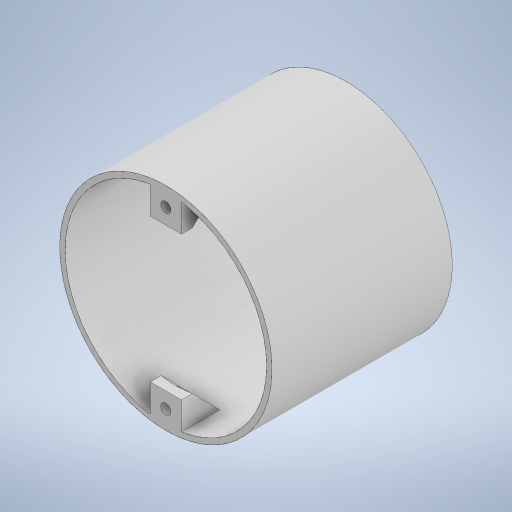
# Autodesk Inventor part: LensMount_mount
Saved by Autodesk Inventor 2023 (Build 270158000, 158)
## iProperties
Created: 2022-10-30
Part Number: LensMount_mount
Material: Generic
Document SubType Name: Modeling
Designer: Piotr
Density: 1 g/cm^3
Appearance: Default
Author: Piotr
Autodesk Inventor part; units mm, degrees
ref_plane "YZ Plane" through (0, 0, 0) normal (1, 0, 0) x (0, 1, 0)
ref_plane "XZ Plane" through (0, 0, 0) normal (0, 1, 0) x (-1, 0, 0)
sketch "Sketch1" plane through (0, 0, 0) normal (0, 0, 1) x (1, 0, 0)
  circle A0 centre (0, 0) radius 32.25
  circle A1 centre (0, 0) radius 34
  line L0 (0, 0) -> (34, 0) construction
  line L1 (0, 0) -> (30.0202, 15.962) construction
  circle A2 centre (0, 0) radius 30.7
  line L2 (0, 0) -> (26.7199, 15.1174) construction
  line L3 (0, 0) -> (27.4745, 13.6983) construction
  line L4 (28.069, 15.8807) -> (29.5921, 16.7424) construction
  line L5 (28.8616, 14.3899) -> (30.4278, 15.1707) construction
  line L6 (27.4745, 13.6983) -> (28.8616, 14.3899)
  line L7 (26.7199, 15.1174) -> (28.069, 15.8807)
  line L8 (-26.7199, -15.1174) -> (-28.069, -15.8807)
  line L9 (-27.4745, -13.6983) -> (-28.8616, -14.3899)
  point P0 (-28.069, -15.8807)
  point P1 (-27.4745, -13.6983)
  dimension "d0" = 64.5
  dimension "d1" = 68
  dimension "d2" = 28
  dimension "d3" = 61.4
  dimension "d4" = 3
  dimension "d11" = 360
  constraints: 20 end point, 7 point on circle, 4 collinear, 3 centre point, 3 coincident, 1 horizontal, 1 symmetric about line, 13 other
  measures "d0" diameter of A0
  measures "d1" diameter of A1
  measures "d2" angle of L0 L1
  measures "d3" diameter of A2
  measures "d4" angle of L3 L2
extrude "Extrusion1" add sketch "Sketch1" along normal blind 1.5 contours L6 A2 L7 A0 | A0 L9 A2 L8 | A1
sketch "Sketch2" plane through (0, 0, 0) normal (0, 0, -1) x (-1, 0, 0)
  line L0 (-27.4745, 13.6983) -> (-28.8616, 14.3899) projected
  arc A0 (-28.8616, 14.3899) -> (28.069, -15.8807) centre (0, 0) ccw projected
  line L1 (28.069, -15.8807) -> (26.7199, -15.1174) projected
  arc A1 (26.7199, -15.1174) -> (27.4745, -13.6983) centre (0, 0) ccw projected
  line L2 (27.4745, -13.6983) -> (28.8616, -14.3899) projected
  arc A2 (28.8616, -14.3899) -> (-28.069, 15.8807) centre (0, 0) ccw projected
  line L3 (-28.069, 15.8807) -> (-26.7199, 15.1174) projected
  arc A3 (-26.7199, 15.1174) -> (-27.4745, 13.6983) centre (0, 0) ccw projected
  circle A4 centre (0, 0) radius 34 projected
  line L4 (0, 0) -> (-34, 0) construction
  arc A5 (-30.7, 0) -> (-29.8518, -7.1668) centre (0, 0) ccw
  arc A6 (-28.9137, -12.8732) -> (-30.0144, -10.0427) centre (0, 0) ccw construction
  line L5 (0, 0) -> (-28.0458, -12.4868) construction
  line L6 (-28.0458, -12.4868) -> (-28.5026, -12.6902) construction
  line L7 (0, 0) -> (-30.0144, -10.0427) construction
  line L8 (0, 0) -> (-30.7755, -7.3885) construction
  line L9 (-30.0144, -10.0427) -> (-29.8518, -7.1668)
  arc A7 (-23.1861, -20.8769) -> (-28.5026, -12.6902) centre (0, 0) ccw construction
  line L10 (0, 0) -> (-23.9664, -21.5795) construction
  line L11 (-28.5026, -12.6902) -> (-28.9137, -12.8732)
  line L12 (0, 0) -> (-19.8551, -25.4133) construction
  line L13 (-23.1861, -20.8769) -> (-19.8551, -25.4133)
  arc A8 (-30.0144, -10.0427) -> (-28.9137, -12.8732) centre (0, 0) ccw
  arc A9 (-28.5026, -12.6902) -> (-23.1861, -20.8769) centre (0, 0) ccw
  arc A10 (-27.4745, 13.6983) -> (-30.7, 0) centre (0, 0) ccw
  arc A11 (-29.8518, -7.1668) -> (-26.7199, 15.1174) centre (0, 0) ccw construction
  arc A12 (-26.7199, 15.1174) -> (-27.4745, 13.6983) centre (0, 0) ccw
  arc A13 (26.7199, -15.1174) -> (27.4745, -13.6983) centre (0, 0) ccw
  arc A14 (27.4745, -13.6983) -> (30.7, 0) centre (0, 0) ccw
  arc A15 (30.7, 0) -> (29.8518, 7.1668) centre (0, 0) ccw
  line L14 (30.0144, 10.0427) -> (29.8518, 7.1668)
  arc A16 (30.0144, 10.0427) -> (28.9137, 12.8732) centre (0, 0) ccw
  line L15 (28.5026, 12.6902) -> (28.9137, 12.8732)
  arc A17 (28.5026, 12.6902) -> (23.1861, 20.8769) centre (0, 0) ccw
  line L16 (23.1861, 20.8769) -> (19.8551, 25.4133)
  line L17 (0, 0) -> (6.3829, -30.0291) construction
  arc A18 (-28.8616, 14.3899) -> (28.069, -15.8807) centre (0, 0) ccw projected
  arc A19 (6.3829, -30.0291) -> (26.7199, -15.1174) centre (0, 0) ccw
  line L18 (6.3829, -30.0291) -> (6.7052, -31.5453)
  line L19 (0, 0) -> (-6.3829, 30.0291) construction
  line L20 (-6.3829, 30.0291) -> (-6.7052, 31.5453)
  arc A20 (-6.3829, 30.0291) -> (-26.7199, 15.1174) centre (0, 0) ccw
  point P0 (28.0458, 12.4868)
  point P1 (27.4745, -13.6983)
  point P2 (-26.7199, 15.1174)
  dimension "d15" = 63.3
  dimension "d16" = 24
  dimension "d17" = 18.5
  dimension "d18" = 13.5
  dimension "d19" = 62.4
  dimension "d20" = 42
  dimension "d21" = 52
  dimension "d24" = 360
  dimension "d43" = 50
  dimension "d46" = 360
  constraints: 39 point on circle, 36 end point, 15 centre point, 6 coincident, 3 collinear, 3 concentric, 3 point on line, 1 horizontal, 1 horizontal alignment, 61 other
  measures "d15" diameter of A6
  measures "d16" angle of L5 L4
  measures "d17" angle of L7 L4
  measures "d18" angle of L8 L4
  measures "d19" diameter of A7
  measures "d20" angle of L4 L10
  measures "d21" angle of L4 L12
  measures "d43" angle of L12 L17
extrude "Extrusion2" add sketch "Sketch2" along normal blind 1.65 contours A10 A5 L9 A8 L11 A9 L13 A0 L0 | L3 A2 L20 A20 | L18 A19 L1 A0 | A2 L2 A14 A15 L14 A16 L15 A17 L16 | A4
sketch "Sketch4" plane through (0, 0, 1.5) normal (0, 0, 1) x (1, 0, 0)
  circle A0 centre (0, 0) radius 34 projected
  arc A1 (28.069, 15.8807) -> (-28.8616, -14.3899) centre (0, 0) ccw projected
  circle A2 centre (0, 0) radius 32.25
  point P0 (-28.8616, -14.3899)
  constraints: 1 centre point, 1 coincident, 1 concentric
extrude "Extrusion4" add sketch "Sketch4" along normal blind 54.6
sketch "Sketch8" plane through (0, 0, 56.1) normal (0, 0, 1) x (1, 0, 0)
  circle A0 centre (0, 0) radius 32.25 projected
  line L0 (0, 0) -> (0, 32.25) construction
  line L1 (-5, 31.86) -> (-5, 23)
  line L2 (-5, 23) -> (5, 23)
  line L3 (5, 31.86) -> (5, 23)
  circle A1 centre (0, 28) radius 1.6
  point P0 (0, 23)
  point P1 (5, 31.86)
  dimension "d53" = 3.2
  dimension "d54" = 4.25
  dimension "d57" = 5
  dimension "d58" = 5
  constraints: 8 end point, 2 point on circle, 2 symmetric about line, 2 vertical, 1 centre point, 1 midpoint, 1 perpendicular, 1 point on line
  measures "d53" diameter of A1
  measures "d54" distance of L0.end A1.centre
  measures "d57" distance from line of L3 A1.centre
  measures "d58" distance from line of A1.centre L2
extrude "Extrusion8" add sketch "Sketch8" against normal blind 3 contours L3 L2 L1 A0 | A1 picked at (0.0643, 24.1372)
chamfer "Chamfer1" distance 9.25 angle 45 1 edges at (0, 32.25, 53.1)
extrude "Extrusion9" cut sketch "Sketch8" against normal blind 10 contours A1
sketch "Sketch9" plane through (0, 0, 56.1) normal (0, 0, 1) x (1, 0, 0)
  circle A0 centre (0, 28) radius 1.6 projected
  line L0 (2.9, 29.6743) -> (2.9, 26.3257)
  line L1 (2.9, 26.3257) -> (0, 24.6514)
  line L2 (0, 24.6514) -> (-2.9, 26.3257)
  line L3 (-2.9, 26.3257) -> (-2.9, 29.6743)
  line L4 (-2.9, 29.6743) -> (0, 31.3486)
  line L5 (0, 31.3486) -> (2.9, 29.6743)
  point P0 (0, 0)
  dimension "d66" = 5.8
  constraints: 12 end point, 1 coincident, 1 vertical, 13 other
  measures "d66" distance between parallel lines of L0 L3
ref_plane "Work Plane1" through (0, 0, 53.1) normal (0, 0, 1) x (1, 0, 0)
extrude "Extrusion10" cut sketch "Sketch9" against normal blind 10 from surface at -3
mirror "Mirror1" about plane through (0, 0, 0) normal (0, 1, 0) of "Extrusion8", "Extrusion10", "Chamfer1", "Extrusion9"
sketch "Sketch10" plane through (-2.9, -29.6743, 53.1) normal (0, 0, -1) x (-1, 0, 0)
  circle A0 centre (-2.9, 1.6743) radius 1.6 projected
  circle A1 centre (-2.9, 57.6743) radius 1.6 projected
  point P0 (-2.9, 29.6743)
extrude "Extrusion11" add sketch "Sketch10" against normal blind 0.2
equation "\"d58\" = d57"
body "Solid1"
